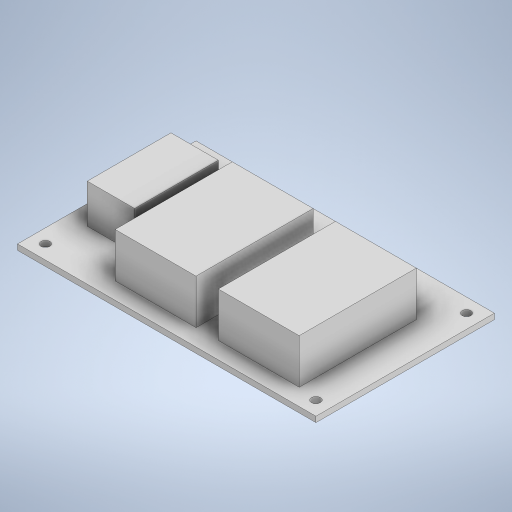
# Autodesk Inventor part: pcb_main_populated
Saved by Autodesk Inventor 2023 (Build 270158000, 158)
## iProperties
Created: 2023-05-10
Part Number: pcb_main_populated
Material: Generic
Document SubType Name: Modeling
Designer: mark
Density: 1 g/cm^3
Appearance: Default
Author: mark
Autodesk Inventor part; units mm, degrees
ref_plane "YZ Plane" through (0, 0, 0) normal (1, 0, 0) x (0, 1, 0)
ref_plane "XZ Plane" through (0, 0, 0) normal (0, 1, 0) x (-1, 0, 0)
ref_plane "XY Plane" through (0, 0, 0) normal (0, 0, 1) x (1, 0, 0)
sketch "Sketch1" plane through (0, 0, 0) normal (0, 1, 0) x (-1, 0, 0)
  line L0 (65.7357, -36.3554) -> (-41.2643, -36.3554)
  line L1 (-41.2643, -36.3554) -> (-41.2643, 27.6446)
  line L2 (-41.2643, 27.6446) -> (65.7357, 27.6446)
  line L3 (65.7357, 27.6446) -> (65.7357, -36.3554)
  circle A0 centre (60.7357, -31.3554) radius 1.6
  circle A1 centre (-36.2643, -31.3554) radius 1.6
  circle A2 centre (60.7357, 22.6446) radius 1.6
  circle A3 centre (-36.2643, 22.6446) radius 1.6
  point P0 (0, 0)
  dimension "d0" = 107
  dimension "d1" = 64
  dimension "d2" = 3.2
  dimension "d3" = 5
  dimension "d4" = 5
  dimension "d7" = 97
  dimension "d10" = 54
  constraints: 8 end point, 4 centre point, 2 horizontal, 2 parallel, 1 perpendicular, 1 vertical, 6 other
  measures "d0" distance of L1.end L2.end
  measures "d1" distance of L0.end L1.end
  measures "d2" diameter of A0
  measures "d3" distance from line of A0.centre L0
  measures "d4" distance from line of L3 A0.centre
  measures "d7" distance of A0.centre A1.centre
  measures "d10" distance of A0.centre A2.centre
extrude "Extrusion1" add sketch "Sketch1" along normal blind 2
sketch "Sketch2" plane through (0, 2, 0) normal (0, 1, 0) x (1, 0, 0)
  line L0 (29.2643, -21.6446) -> (0.2643, -21.6446)
  line L1 (0.2643, -21.6446) -> (0.2643, 20.3554)
  line L2 (0.2643, 20.3554) -> (29.2643, 20.3554)
  line L3 (29.2643, 20.3554) -> (29.2643, -21.6446)
  line L4 (41.2643, -27.6446) -> (41.2643, 36.3554) projected
  line L5 (-65.7357, -27.6446) -> (41.2643, -27.6446) projected
  line L6 (-36.7357, -21.6446) -> (-36.7357, 20.3554)
  line L7 (-36.7357, 20.3554) -> (-7.7357, 20.3554)
  line L8 (-7.7357, 20.3554) -> (-7.7357, -21.6446)
  line L9 (-7.7357, -21.6446) -> (-36.7357, -21.6446)
  point P0 (0, 0)
  dimension "d15" = 29
  dimension "d16" = 42
  dimension "d17" = 12
  dimension "d18" = 6
  dimension "d21" = 37
  constraints: 16 end point, 2 horizontal, 2 parallel, 1 perpendicular, 8 other
  measures "d15" distance of L1.end L2.end
  measures "d16" distance of L0.end L1.end
  measures "d17" distance between parallel lines of L4 L3
  measures "d18" distance between parallel lines of L5 L0
  measures "d21" distance of L0.end L6.start
extrude "Extrusion2" add sketch "Sketch2" along normal blind 16
sketch "Sketch3" plane through (0, 2, 0) normal (0, 1, 0) x (1, 0, 0)
  line L0 (-58.7357, 20.3554) -> (-41.7357, 20.3554)
  line L1 (-41.7357, 20.3554) -> (-41.7357, -9.6446)
  line L2 (-41.7357, -9.6446) -> (-58.7357, -9.6446)
  line L3 (-58.7357, -9.6446) -> (-58.7357, 20.3554)
  line L4 (-7.7357, 20.3554) -> (-36.7357, 20.3554) projected
  line L5 (-36.7357, 20.3554) -> (-36.7357, -21.6446) projected
  point P0 (0, 0)
  dimension "d28" = 17
  dimension "d29" = 30
  dimension "d30" = 5
  constraints: 8 end point, 2 parallel, 1 collinear, 1 horizontal, 1 perpendicular
  measures "d28" distance of L1.end L2.end
  measures "d29" distance of L0.end L1.end
  measures "d30" distance between parallel lines of L5 L1
extrude "Extrusion3" add sketch "Sketch3" along normal blind 14
body "Solid1"
